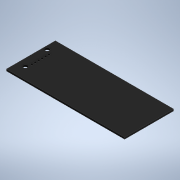
# Autodesk Inventor part: akkum_board
Saved by Autodesk Inventor 2020 (Build 240168000, 168)
## iProperties
Created: 2022-07-19
Part Number: akkum_board
Material: Типовые
Document SubType Name: Modeling
Designer: akapu
Density: 1 g/cm^3
Appearance: По умолчанию
Author: akapu
Autodesk Inventor part; units mm, degrees
ref_plane "YZ Plane" through (0, 0, 0) normal (1, 0, 0) x (0, 1, 0)
ref_plane "XZ Plane" through (0, 0, 0) normal (0, 1, 0) x (-1, 0, 0)
ref_plane "XY Plane" through (0, 0, 0) normal (0, 0, 1) x (1, 0, 0)
sketch "Эскиз1" plane through (0, 0, 0) normal (0, 1, 0) x (-1, 0, 0)
  line L0 (-5.5, -11.8) -> (-4.75, -11.8)
  circle A0 centre (-4.75, -8.8) radius 1.25
  circle A1 centre (-2.5, -23.8) radius 1.25
  circle A2 centre (-5.5, -19.8) radius 0.6
  circle A3 centre (-5.5, -21.8) radius 0.6
  circle A4 centre (-5.5, -17.8) radius 0.6
  circle A5 centre (-5.5, -15.8) radius 0.6
  circle A6 centre (-5.5, -13.8) radius 0.6
  circle A7 centre (-5.5, -11.8) radius 0.6
  line L1 (-0.5, -32.6) -> (-0.5, 0)
  line L2 (-0.5, -32.6) -> (-0.5, 0)
  line L3 (-0.5, 0) -> (-67.5, 0)
  line L4 (-67.5, 0) -> (-67.5, -32.6)
  line L5 (-67.5, -32.6) -> (-0.5, -32.6)
  line L6 (-0.5, -32.6) -> (-0.5, 0)
  dimension "d37" = 2.5
  dimension "d39" = 1.2
  dimension "d40" = 1.2
  dimension "d41" = 1.2
  dimension "d42" = 1.2
  dimension "d43" = 1.2
  dimension "d44" = 1.2
  dimension "d47" = 67
  constraints: 14 end point, 8 centre point, 2 horizontal, 2 parallel, 1 coincident, 1 perpendicular
  measures "d37" diameter of A0
  measures "d39" diameter of A2
  measures "d40" diameter of A3
  measures "d41" diameter of A4
  measures "d42" diameter of A5
  measures "d43" diameter of A6
  measures "d44" diameter of A7
  measures "d47" distance of L5.end L4.end
extrude "Выдавливание1" add sketch "Эскиз1" along normal blind 1
sketch "Эскиз2" plane through (0, 1, 0) normal (0, 1, 0) x (1, 0, 0)
  line L0 (0.5, 0) -> (67.5, 0) projected
  line L1 (0.5, 0) -> (0.5, 2)
  line L2 (0.5, 32.6) -> (0.5, 0) projected
  line L3 (0.5, 2) -> (67.5, 2)
  line L4 (67.5, 0) -> (67.5, 32.6) projected
  line L5 (0.5, 32.6) -> (0.5, 30.6)
  line L6 (0.5, 30.6) -> (67.5, 30.6)
  line L7 (67.5, 30.6) -> (68.5, 30.6)
  line L8 (68.5, 30.6) -> (68.5, 2)
  line L9 (68.5, 2) -> (67.5, 2)
  line L10 (67.5, 32.6) -> (0.5, 32.6) projected
  line L11 (0.5, 0) -> (67.5, 0)
  line L12 (67.5, 0) -> (67.5, 32.6)
  line L13 (67.5, 32.6) -> (0.5, 32.6)
  line L14 (0.5, 32.6) -> (0.5, 0)
  point P0 (0, 0)
  dimension "d48" = 2
  dimension "d49" = 2
  dimension "d50" = 1
  constraints: 22 end point, 5 perpendicular, 5 point on line, 2 parallel, 1 horizontal
  measures "d48" distance of L0.start L1.end
  measures "d49" distance of L2.start L5.end
  measures "d50" distance of L6.end L7.end
extrude "Выдавливание2" cut sketch "Эскиз2" against normal blind 10 contours L1 L3 L4 L0 | L2 L10 L4 L6
sketch "Эскиз3" plane through (0, 1, 0) normal (0, 1, 0) x (1, 0, 0)
  line L0 (67.5, 2) -> (67.5, 30.6) projected
  line L1 (67.5, 2) -> (69.5, 2)
  line L2 (69.5, 2) -> (69.5, 30.6)
  line L3 (69.5, 30.6) -> (67.5, 30.6)
  line L4 (67.5, 30.6) -> (67.5, 2)
  point P0 (0, 0)
  dimension "d53" = 2
  constraints: 8 end point, 2 parallel, 1 horizontal, 1 perpendicular
  measures "d53" distance of L3.end L2.end
extrude "Выдавливание3" add sketch "Эскиз3" against normal blind 1
